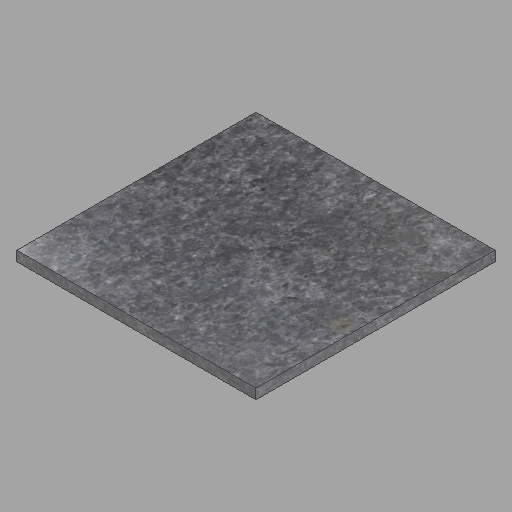
# Autodesk Inventor part: 24x24x2-75
Saved by Autodesk Inventor 2023 (Build 270158000, 158)
## iProperties
Created: 2022-03-01
Part Number: 24x24x2-75
Material: Granite, Cut, Polished
Document SubType Name: Modeling
Designer: awelt
Mass: 25485.2 g
Surface Area: 8051.6 cm^2
Volume: 9438.95 cm^3
Density: 2.7 g/cm^3
Appearance: Kasota SN sapphire
TEST: 0.0
Author: awelt
Autodesk Inventor part; units mm, degrees
ref_plane "YZ Plane" through (0, 0, 0) normal (1, 0, 0) x (0, 1, 0)
ref_plane "XZ Plane" through (0, 0, 0) normal (0, 1, 0) x (-1, 0, 0)
ref_plane "XY Plane" through (0, 0, 0) normal (0, 0, 1) x (1, 0, 0)
sketch "Sketch1" plane through (0, 0, 0) normal (0, 1, 0) x (-1, 0, 0)
  line L0 (304.8, -304.8) -> (-304.8, -304.8)
  line L1 (-304.8, -304.8) -> (-304.8, 304.8)
  line L2 (-304.8, 304.8) -> (304.8, 304.8)
  line L3 (304.8, 304.8) -> (304.8, -304.8)
  line L4 (304.8, -304.8) -> (-304.8, 304.8) construction
  line L5 (-304.8, -304.8) -> (304.8, 304.8) construction
  point P0 (0, 0)
  dimension "d0" = 609.6
  dimension "d1" = 609.6
  constraints: 12 end point, 2 midpoint, 2 parallel, 1 horizontal, 1 perpendicular
  measures "d0" distance of L1.end L2.end
  measures "d1" distance of L0.end L1.end
extrude "Extrusion1" add sketch "Sketch1" along normal blind 25.4
body "Solid1"
